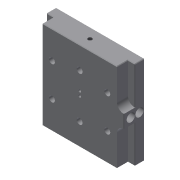
# Autodesk Inventor part: bottomplate
Saved by Autodesk Inventor 2022 (Build 260148000, 148)
## iProperties
Shininess: 64.0
Length Units: 11272
Angle Units: 11279
Time Units: 11290
Mass Units: 11286
Length Display Precision: 3
Angle Display Precision: 2
Compacted: True
Part Number: bottomplate
Document SubType Name: Modeling
Created: 2003-04-04
Designer: demo
Density: 1 g/cm^3
Material: Generic
Appearance: Default
Density: 0.0
Volumn: 0.0
Area: 0.0
PropertySet Name: Model Information
Control State: 0
Master: False
Checked Out: False
Author: demo
Autodesk Inventor part; units mm, degrees
sketch "Sketch1" plane through (0, 0, 0) normal (0, 0, 1) x (1, 0, 0)
  line L0 (-8.6563, -172.2568) -> (194.5437, -172.2568)
  line L1 (194.5437, -172.2568) -> (194.5437, 30.9432)
  line L2 (194.5437, 30.9432) -> (-8.6563, 30.9432)
  line L3 (-8.6563, 30.9432) -> (-8.6563, -172.2568)
  dimension "d0" = 203.2
  dimension "d1" = 203.2
  constraints: 8 end point, 2 parallel, 1 horizontal, 1 perpendicular
  measures "d0" distance of L1.end L2.end
  measures "d1" distance of L2.end L0.start
extrude "Extrusion1" add sketch "Sketch1" along normal blind 47.625
sketch "Sketch2" plane through (0, 0, 47.625) normal (0, 0, 1) x (1, 0, 0)
  line L0 (-8.6563, -172.2568) -> (-8.6563, 30.9432) projected
  line L1 (7.2187, -172.2568) -> (7.2187, 30.9432)
  line L2 (-8.6563, 30.9432) -> (7.2187, 30.9432)
  line L3 (-8.6563, -172.2568) -> (7.2187, -172.2568)
  dimension "d4" = 15.875
  constraints: 6 end point, 1 parallel, 1 perpendicular
  measures "d4" distance between parallel lines of L1 L0
extrude "Extrusion2" cut sketch "Sketch2" against normal blind 25.273
sketch "Sketch3" plane through (0, 0, 47.625) normal (0, 0, 1) x (1, 0, 0)
  line L0 (194.5437, -172.2568) -> (7.2187, -172.2568) projected
  line L1 (194.5437, 30.9432) -> (194.5437, -172.2568) projected
  line L2 (7.2187, 30.9432) -> (194.5437, 30.9432) projected
  line L3 (178.6687, -172.2568) -> (178.6687, -100.8828)
  line L4 (193.9087, -85.6428) -> (194.5437, -85.6428)
  arc A0 (193.9087, -85.6428) -> (178.6687, -100.8828) centre (193.9087, -100.8828) ccw
  point P0 (178.6687, -85.6428)
  dimension "d7" = 86.614
  dimension "d8" = 15.875
  dimension "d9" = 15.24
  constraints: 4 end point, 4 point on line, 2 perpendicular, 2 point on circle, 2 tangent, 1 centre point
  measures "d7" distance of L3.start point (178.669, -85.643)
  measures "d8" distance of L0.start L3.start
  measures "d9" radius of A0
extrude "Extrusion3" cut sketch "Sketch3" against normal blind 25.273
ref_plane "Work Plane1" through (-8.6563, -70.6568, 0) normal (0, 1, 0) x (1, 0, 0)
mirror "Mirror1" about plane through (-8.6563, -70.6568, 0) normal (0, 1, 0) of "Extrusion3"
ref_plane "Work Plane2" through (92.9437, -172.2568, 0) normal (1, 0, 0) x (0, 0, -1)
sketch "Sketch4" plane through (6.3634, 2.4807, 0) normal (0, 0, -1) x (-1, 0, 0)
  line L0 (-188.2129, -174.324) -> (-188.2129, -101.299)
  line L1 (14.9871, -174.324) -> (-188.2129, -174.324)
  line L2 (-86.6129, -194.644) -> (-86.6129, 89.836)
  line L3 (-249.1729, -72.724) -> (35.3071, -72.724)
  point P0 (-86.6129, -123.524)
  point P1 (-150.1129, -110.824)
  point P2 (-23.1129, -110.824)
  point P3 (-150.1129, -34.624)
  point P4 (-23.1129, -34.624)
  point P5 (-86.6129, -21.924)
  dimension "d15" = 50.8
  dimension "d14" = 38.1
  dimension "d13" = 63.5
  constraints: 8 end point, 4 symmetric about line, 1 point on line
  measures "d15" distance from line of L1 point (-86.613, -123.524)
  measures "d14" distance from line of L0 point (-150.113, -110.824)
  measures "d13" distance from line of L1 point (-150.113, -110.824)
hole "Hole1" at (92.9763, -121.0433, 0) at (156.4763, -108.3433, 0) at (29.4763, -108.3433, 0) at (156.4763, -32.1433, 0) at (29.4763, -32.1433, 0) at (92.9763, -19.4433, 0) direction (0, 0, 1) diameter 13.4925 end through all counterbore diameter 19.8425 counterbore depth 15.875
ref_plane "Work Plane3" through (0, 0, 23.8125) normal (0, 0, 1) x (1, 0, 0)
sketch "Sketch5" plane through (-8.6563, -172.2568, 0) normal (0, -1, 0) x (1, 0, 0)
  line L0 (187.325, 47.625) -> (15.875, 47.625) projected
  line L1 (101.6, 61.9125) -> (101.6, -4.7625) projected
  point P0 (101.6, 23.8252)
  dimension "d22" = 23.7998
  constraints: 1 point on line
  measures "d22" distance from line of L0 point (101.6, 23.825)
hole "Hole2" at (92.9437, -172.2568, 23.8252) direction (0, 1, 0) diameter 9.144 depth 26.1112 tip angle 118 thread size "7/16-14 UNC" class "1B" standard "ANSI Unified Screw Threads"
mirror "Mirror2" about plane through (-8.6563, -70.6568, 0) normal (0, 1, 0) of "Hole2"
sketch "Sketch6" plane through (194.5437, -172.2568, 0) normal (1, 0, 0) x (0, 0, -1)
  line L0 (-22.352, 116.586) -> (-47.625, 116.586) projected
  line L1 (-47.625, 116.586) -> (-47.625, 86.614) projected
  point P0 (-31.75, 101.4984)
  dimension "d30" = 15.875
  dimension "d31" = 15.0876
  measures "d30" distance from line of L1 point (-31.75, 101.498)
  measures "d31" distance from line of L0 point (-31.75, 101.498)
hole "Hole3" at (194.5437, -70.7584, 31.75) direction (-1, 0, 0) diameter 9.144 depth 102.235 tip angle 118 counterbore diameter 19.05 counterbore depth 17.4625 thread size "7/16-14 UNC" class "1B" standard "ANSI Unified Screw Threads"
sketch "Sketch7" plane through (194.5437, -172.2568, 0) normal (1, 0, 0) x (0, 0, -1)
  line L0 (-47.625, 86.614) -> (-22.352, 86.614) projected
  line L1 (0, 0) -> (0, 203.2) projected
  point P0 (-11.684, 101.6)
  dimension "d39" = 14.986
  dimension "d40" = 11.684
  measures "d39" distance from line of L0 point (-11.684, 101.6)
  measures "d40" distance from line of L1 point (-11.684, 101.6)
hole "Hole4" at (194.5437, -70.6568, 11.684) direction (-1, 0, 0) diameter 9.144 depth 102.235 tip angle 118 counterbore diameter 19.05 counterbore depth 17.4625 thread size "7/16-14 UNC" class "1B" standard "ANSI Unified Screw Threads"
sketch "Sketch8" plane through (0, 0, 47.625) normal (0, 0, 1) x (1, 0, 0)
  line L0 (-28.9763, -70.6568) -> (255.5037, -70.6568) projected
  line L1 (92.9437, 91.9032) -> (92.9437, -192.5768) projected
  point P0 (92.9437, -70.6568)
  constraints: 2 point on line
hole "Hole5" at (92.9437, -70.6568, 47.625) direction (0, 0, -1) diameter 6.35 depth 38.5064 tip angle 118
sketch "Sketch9" plane through (0, 0, 47.625) normal (0, 0, 1) x (1, 0, 0)
  circle A0 centre (92.9437, -70.6568) radius 3.175 projected
  point P0 (92.9437, -60.3444)
  dimension "d55" = 10.3124
  measures "d55" distance of A0.centre point (92.944, -60.344)
hole "Hole6" at (92.9437, -60.3444, 47.625) direction (0, 0, -1) diameter 6.35 depth 38.5064 tip angle 118
chamfer "Chamfer1" distance 1.27 angle 45 23 edges at (7.2187, -70.6568, 47.625) (92.9437, 30.9432, 47.625) (92.9437, -172.2568, 47.625) (194.5437, -70.6568, 47.625) (194.5437, -128.9498, 22.352) (178.6687, -172.2568, 34.9885) (186.6062, -172.2568, 22.352) (194.5437, -172.2568, 11.176) (194.5437, -70.6568, 0) (194.5437, -12.3638, 22.352) (194.5437, 30.9432, 11.176) (186.6062, 30.9432, 22.352) (178.6687, 30.9432, 34.9885) (7.2187, 30.9432, 34.9885) (-0.7188, 30.9432, 22.352) (-8.6563, -70.6568, 22.352) (7.2187, -172.2568, 34.9885) (-0.7188, -172.2568, 22.352) (92.9437, 30.9432, 0) (-8.6563, 30.9432, 11.176) (-8.6563, -70.6568, 0) (92.9437, -172.2568, 0) (-8.6563, -172.2568, 11.176)
body "Solid1"
